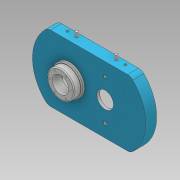
# Autodesk Inventor part: 밑판(new)
Saved by Autodesk Inventor 2018 (Build 220112000, 112)
## iProperties
Created: 2018-04-19
Part Number: 밑판(new)
Material: 일반
Document SubType Name: Modeling
Designer: CK
Density: 1 g/cm^3
Appearance: 기본값
Author: CK
Autodesk Inventor part; units mm, degrees
ref_plane "YZ Plane" through (0, 0, 0) normal (1, 0, 0) x (0, 1, 0)
ref_plane "XZ Plane" through (0, 0, 0) normal (0, 1, 0) x (-1, 0, 0)
ref_plane "XY Plane" through (0, 0, 0) normal (0, 0, 1) x (1, 0, 0)
sketch "스케치1" plane through (0, 0, 0) normal (0, 1, 0) x (-1, 0, 0)
  line L0 (-45, 36) -> (45, 36)
  line L1 (45, 36) -> (45, -36)
  line L2 (45, -36) -> (-45, -36)
  line L3 (-45, -36) -> (-45, 36)
  line L4 (-45, 36) -> (45, -36) construction
  line L5 (45, 36) -> (-45, -36) construction
  arc A0 (45, -36) -> (45, 36) centre (14.0366, 0) ccw
  line L6 (0, 68.3941) -> (0, -86.625) construction
  arc A1 (-45, 36) -> (-45, -36) centre (-14.0366, 0) ccw
  point P0 (0, 0)
  dimension "d0" = 90
  dimension "d1" = 72
  constraints: 14 end point, 4 point on circle, 2 centre point, 2 midpoint, 2 parallel, 1 horizontal, 1 perpendicular, 1 symmetric about line, 1 vertical, 1 other
  measures "d0" distance of L1.end L2.end
  measures "d1" distance of L0.end L1.end
extrude "돌출1" add sketch "스케치1" along normal blind 12
fillet "모깎기1" radius 8 4 edges at (45, 6, 36) (-45, 6, 36) (-45, 6, -36) (45, 6, -36)
shell "쉘1" thickness 5 removed faces 1 at (-13.9584, 12, 12)
sketch "스케치2" plane through (0, 0, 0) normal (0, -1, 0) x (1, 0, 0)
  circle A0 centre (-21, 0) radius 15
  circle A1 centre (-21, 0) radius 16.25
  point P0 (0, 0)
  dimension "d6" = 21
  dimension "d7" = 30
  dimension "d8" = 32.5
  constraints: 2 centre point, 1 coincident
  measures "d6" distance of A0.centre point (0, 0)
  measures "d7" diameter of A0
  measures "d8" diameter of A1
extrude "돌출2" add sketch "스케치2" along normal blind 3 contours A0 | A1
sketch "스케치3" plane through (-21, -3, 0) normal (0, -1, 0) x (1, 0, 0)
  circle A0 centre (0, 0) radius 14.75
  point P0 (21, 0)
  dimension "d11" = 29.5
  constraints: 1 centre point
  measures "d11" diameter of A0
extrude "돌출3" add sketch "스케치3" along normal blind 7
sketch "스케치4" plane through (-21, -10, 0) normal (0, -1, 0) x (1, 0, 0)
  circle A0 centre (0, 0) radius 9
  point P0 (21, 0)
  dimension "d14" = 18
  constraints: 1 centre point
  measures "d14" diameter of A0
extrude "돌출4" cut sketch "스케치4" against normal through all
fillet "모깎기2" radius 1 1 edges at (-35.75, -10, 0)
sketch "스케치5" plane through (0, 0, 0) normal (0, -1, 0) x (1, 0, 0)
  circle A0 centre (-21, 0) radius 9 projected
  circle A1 centre (17.5, 0) radius 9
  point P0 (0, 0)
  dimension "d18" = 18
  dimension "d19" = 38.5
  constraints: 1 centre point
  measures "d18" diameter of A1
  measures "d19" distance of A0.centre A1.centre
extrude "돌출5" cut sketch "스케치5" against normal blind 10 contours A1
sketch "스케치6" plane through (-21, -10, 0) normal (0, -1, 0) x (1, 0, 0)
  circle A0 centre (0, 0) radius 12 construction
  circle A1 centre (-12, 0) radius 0.9
  point P0 (21, 0)
  dimension "d22" = 24
  dimension "d23" = 1.8
  constraints: 1 centre point, 1 horizontal alignment, 2 other
  measures "d23" diameter of A1
extrude "돌출6" cut sketch "스케치6" against normal blind 5
pattern_circular "원형 패턴1" count 6 over 360 about axis through (-21, -10, 0) along (0, 1, 0) of "돌출6"
sketch "스케치7" plane through (0, 0, 0) normal (0, -1, 0) x (1, 0, 0)
  circle A0 centre (17.5, 0) radius 9 projected
  circle A1 centre (17.5, 21.915) radius 1.5
  circle A2 centre (17.5, -21.915) radius 2
  point P0 (0, 0)
  dimension "d29" = 3
  dimension "d30" = 21.915
  dimension "d31" = 4
  dimension "d32" = 21.915
  constraints: 2 centre point
  measures "d29" diameter of A1
  measures "d30" distance of A0.centre A1.centre
  measures "d31" diameter of A2
  measures "d32" distance of A2.centre A0.centre
extrude "돌출7" cut sketch "스케치7" against normal blind 7 contours A1 | A2
sketch "스케치9" plane through (-41.8752, 0, 36) normal (0, 0, 1) x (1, 0, 0)
  line L0 (-3.3551, 8) -> (110.2379, 8) construction
  line L1 (0, 0) -> (83.7504, 0) projected
  line L2 (20.3752, 11.2841) -> (20.3752, -22.7562) construction
  line L3 (10.3752, 14.1991) -> (10.3752, -23.7906) construction
  line L4 (41.8752, 0) -> (41.8752, 28.3042) construction
  line L5 (63.3752, 11.2841) -> (63.3752, -22.7562) construction
  line L6 (73.3752, 14.1991) -> (73.3752, -23.7906) construction
  circle A0 centre (20.3752, 8) radius 1.5
  circle A1 centre (63.3752, 8) radius 1.5
  dimension "d39" = 8
  dimension "d40" = 31.5
  dimension "d41" = 21.5
  dimension "d42" = 3
  dimension "d43" = 3
  constraints: 12 end point, 4 point on line, 4 symmetric about line, 3 vertical, 2 centre point, 1 horizontal
  measures "d39" distance between parallel lines of L1 L0
  measures "d40" distance from line of L4.start L3
  measures "d41" distance from line of L4.start L2
  measures "d42" diameter of A0
  measures "d43" diameter of A1
extrude "돌출9" add sketch "스케치9" along normal blind 5
sketch "스케치10" plane through (-41.8752, 0, 36) normal (0, 0, 1) x (1, 0, 0)
  line L0 (-42.2154, 8) -> (125.0102, 8) construction
  line L1 (10.3752, 32.8081) -> (10.3752, -49.6899)
  line L2 (73.3752, 21.1819) -> (73.3752, -27.2339)
  circle A0 centre (10.3752, 8) radius 1.25
  circle A1 centre (73.3752, 8) radius 1.25
  point P0 (41.8752, 0)
  dimension "d46" = 8
  dimension "d47" = 31.5
  dimension "d48" = 31.5
  dimension "d49" = 2.5
  dimension "d50" = 2.5
  constraints: 6 end point, 4 point on line, 2 centre point, 2 vertical, 1 horizontal
  measures "d46" distance from line of point (41.875, 0) L0
  measures "d47" distance from line of point (41.875, 0) L1
  measures "d48" distance from line of L2 point (41.875, 0)
  measures "d49" diameter of A0
  measures "d50" diameter of A1
extrude "돌출10" cut sketch "스케치10" against normal blind 8.8
fillet "모깎기3" radius 1 1 edges at (-37.25, -3, 0)
mirror "미러2" about plane through (0, 0, 0) normal (0, 0, 1) of "돌출10", "돌출9"
sketch "스케치12" plane through (-14.0366, 5, 0) normal (0, 1, 0) x (1, 0, 0)
  arc A0 (-29.9538, 30.1274) -> (-29.9538, -30.1274) centre (0, 0) ccw projected
  arc A1 (-27.8386, 31) -> (-29.9538, 30.1274) centre (-27.8386, 28) ccw projected
  line L0 (-27.8386, 31) -> (55.9118, 31) projected
  arc A2 (58.0269, 30.1274) -> (55.9118, 31) centre (55.9118, 28) ccw projected
  arc A3 (58.0269, -30.1274) -> (58.0269, 30.1274) centre (28.0731, 0) ccw projected
  arc A4 (55.9118, -31) -> (58.0269, -30.1274) centre (55.9118, -28) ccw projected
  line L1 (55.9118, -31) -> (-27.8386, -31) projected
  arc A5 (-29.9538, -30.1274) -> (-27.8386, -31) centre (-27.8386, -28) ccw projected
  point P0 (14.0366, 0)
extrude "돌출12" cut sketch "스케치12" against normal blind 2
sketch "스케치14" plane through (-14.0366, 3, 0) normal (0, 1, 0) x (1, 0, 0)
  arc A0 (-17.9634, -8.6603) -> (-17.9634, 8.6603) centre (-6.9634, 0) ccw
  line L0 (-17.9634, -8.6603) -> (-17.9634, 8.6603)
  point P0 (14.0366, 0)
  dimension "d62" = 28
  dimension "d63" = 25
  constraints: 2 end point, 2 point on circle, 1 centre point, 1 coincident, 1 vertical
  measures "d62" diameter of A0
extrude "돌출14" cut sketch "스케치14" against normal blind 3
